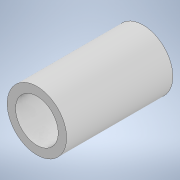
# Autodesk Inventor part: 1_5 inch PVC Spacer
Saved by Autodesk Inventor 2020 (Build 240168000, 168)
## iProperties
Created: 2020-02-01
Part Number: 1_5 inch PVC Spacer
Material: Generic
Document SubType Name: Modeling
Designer: JimAndVal
Density: 1 g/cm^3
Appearance: Default
Author: JimAndVal
Autodesk Inventor part; units mm, degrees
ref_plane "YZ Plane" through (0, 0, 0) normal (1, 0, 0) x (0, 1, 0)
ref_plane "XZ Plane" through (0, 0, 0) normal (0, 1, 0) x (-1, 0, 0)
ref_plane "XY Plane" through (0, 0, 0) normal (0, 0, 1) x (1, 0, 0)
sketch "Sketch1" plane through (0, 0, 0) normal (0, 0, 1) x (1, 0, 0)
  circle A0 centre (0, 0) radius 7.6454
  circle A1 centre (0, 0) radius 10.668
  dimension "d0" = 15.2908
  dimension "d1" = 21.336
  constraints: 2 centre point, 2 coincident
  measures "d0" diameter of A0
  measures "d1" diameter of A1
extrude "Extrusion1" add sketch "Sketch1" along normal mid plane 38.1
body "Solid1"
